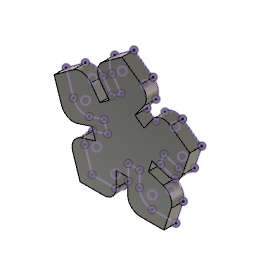
pentagon (Autodesk Fusion 360 design; units mm, degrees)
Autodesk Fusion 360 part; units mm, degrees
sketch "Sketch1" plane through (0, 0, 0) normal (0, 1, 0) x (1, 0, 0)
  line L0 (0, 10.6457) -> (2.025, 10.6457)
  line L1 (2.025, 10.6457) -> (2.025, 20.6457)
  line L2 (-2.025, 10.6457) -> (-2.025, 20.6457)
  line L3 (0, 10.6457) -> (-2.025, 10.6457)
  line L4 (-9.4989, 5.2156) -> (-19.0095, 8.3058)
  line L5 (-10.7504, 1.3638) -> (-20.261, 4.454)
  line L6 (-10.1247, 3.2897) -> (-10.7504, 1.3638)
  line L7 (-10.1247, 3.2897) -> (-9.4989, 5.2156)
  line L8 (-7.8957, -7.4223) -> (-13.7735, -15.5125)
  line L9 (-4.6191, -9.8028) -> (-10.497, -17.893)
  line L10 (-6.2574, -8.6126) -> (-4.6191, -9.8028)
  line L11 (-6.2574, -8.6126) -> (-7.8957, -7.4223)
  line L12 (4.6191, -9.8028) -> (10.497, -17.893)
  line L13 (7.8957, -7.4223) -> (13.7735, -15.5125)
  line L14 (6.2574, -8.6126) -> (7.8957, -7.4223)
  line L15 (6.2574, -8.6126) -> (4.6191, -9.8028)
  line L16 (10.7504, 1.3638) -> (20.261, 4.454)
  line L17 (9.4989, 5.2156) -> (19.0095, 8.3058)
  line L18 (10.1247, 3.2897) -> (9.4989, 5.2156)
  line L19 (10.1247, 3.2897) -> (10.7504, 1.3638)
  line L20 (-24.2705, -7.886) -> (-13.7735, -15.5125)
  line L21 (-10.497, -17.893) -> (0, -25.5195)
  line L22 (-15, 20.6457) -> (-19.0095, 8.3058)
  line L23 (-20.261, 4.454) -> (-24.2705, -7.886)
  line L24 (15, 20.6457) -> (2.025, 20.6457)
  line L25 (-2.025, 20.6457) -> (-15, 20.6457)
  line L26 (24.2705, -7.886) -> (20.261, 4.454)
  line L27 (19.0095, 8.3058) -> (15, 20.6457)
  line L28 (0, -25.5195) -> (10.497, -17.893)
  line L29 (13.7735, -15.5125) -> (24.2705, -7.886)
  dimension "d9" = 360
  constraint perpendicular L1 L24
  constraint collinear L20 L21
  constraint collinear L22 L23
  constraint collinear L24 L25
  constraint collinear L26 L27
  constraint collinear L28 L29
extrude "Extrude1" add sketch "Sketch1" along normal blind 4.3
fillet "Fillet1" radius 4.5 10 edges at (-2.025, 2.15, -20.6457) (2.025, 2.15, -20.6457) (19.0095, 2.15, -8.3058) (20.261, 2.15, -4.454) (10.497, 2.15, 17.893) (13.7735, 2.15, 15.5125) (-19.0095, 2.15, -8.3058) (-20.261, 2.15, -4.454) (-13.7735, 2.15, 15.5125) (-10.497, 2.15, 17.893)
sketch "Sketch2" plane through (0, 4.3, 0) normal (0, 1, 0) x (-1, 0, 0)
  arc A0 (7.852, 14.2524) -> (6.8564, 20.538) centre (4.2114, 16.8975) ccw
  line L0 (6.8564, 20.538) -> (0, 25.5195)
  line L1 (0, 25.5195) -> (-6.8564, 20.538)
  arc A1 (-6.8564, 20.538) -> (-7.852, 14.2524) centre (-4.2114, 16.8975) ccw
  line L2 (-7.852, 14.2524) -> (-4.6191, 9.8028)
  line L3 (-4.6191, 9.8028) -> (-7.8957, 7.4223)
  line L4 (-7.8957, 7.4223) -> (-11.1285, 11.8719)
  arc A2 (-11.1285, 11.8719) -> (-17.4141, 12.8674) centre (-14.7691, 9.2269) ccw
  line L5 (-17.4141, 12.8674) -> (-24.2705, 7.886)
  line L6 (-24.2705, 7.886) -> (-21.6516, -0.1742)
  arc A3 (-21.6516, -0.1742) -> (-15.9813, -3.0634) centre (-17.3718, 1.2163) ccw
  line L7 (-15.9813, -3.0634) -> (-10.7504, -1.3638)
  line L8 (-10.7504, -1.3638) -> (-9.4989, -5.2156)
  line L9 (-9.4989, -5.2156) -> (-14.7297, -6.9152)
  arc A4 (-14.7297, -6.9152) -> (-17.6189, -12.5855) centre (-13.3392, -11.1949) ccw
  line L10 (-17.6189, -12.5855) -> (-15, -20.6457)
  line L11 (-15, -20.6457) -> (-6.525, -20.6457)
  arc A5 (-6.525, -20.6457) -> (-2.025, -16.1457) centre (-6.525, -16.1457) ccw
  line L12 (-2.025, -16.1457) -> (-2.025, -10.6457)
  line L13 (-2.025, -10.6457) -> (2.025, -10.6457)
  line L14 (2.025, -10.6457) -> (2.025, -16.1457)
  arc A6 (2.025, -16.1457) -> (6.525, -20.6457) centre (6.525, -16.1457) ccw
  line L15 (6.525, -20.6457) -> (15, -20.6457)
  line L16 (15, -20.6457) -> (17.6189, -12.5855)
  arc A7 (17.6189, -12.5855) -> (14.7297, -6.9152) centre (13.3392, -11.1949) ccw
  line L17 (14.7297, -6.9152) -> (9.4989, -5.2156)
  line L18 (9.4989, -5.2156) -> (10.7504, -1.3638)
  line L19 (10.7504, -1.3638) -> (15.9813, -3.0634)
  arc A8 (15.9813, -3.0634) -> (21.6516, -0.1742) centre (17.3718, 1.2163) ccw
  line L20 (21.6516, -0.1742) -> (24.2705, 7.886)
  line L21 (24.2705, 7.886) -> (17.4141, 12.8674)
  arc A9 (17.4141, 12.8674) -> (11.1285, 11.8719) centre (14.7691, 9.2269) ccw
  line L22 (11.1285, 11.8719) -> (7.8957, 7.4223)
  line L23 (7.8957, 7.4223) -> (4.6191, 9.8028)
  line L24 (4.6191, 9.8028) -> (7.852, 14.2524)
equation "thickness = 4.3 mm"
equation "notch_depth = 7 mm"
equation "length = 30 mm"
equation "kerf = 0.25 mm"
equation "d10 = thickness"
